Autodesk Fusion 360 part; units mm, degrees
(part 3 of 3)
  line L0 (23, 63.192) -> (0, 63.192)
  line L1 (0, 63.192) -> (0, 51.1685)
  line L2 (0, 51.1685) -> (23, 51.1685)
  line L3 (23, 51.1685) -> (23, 63.192)
  point P0 (22.9329, 63.145)
  point P1 (22.8659, 63.098)
  point P2 (22.799, 63.0511)
  point P3 (22.7322, 63.0043)
  point P4 (22.6656, 62.9575)
  point P5 (22.5991, 62.9107)
  point P6 (22.5326, 62.864)
  point P7 (22.4664, 62.8174)
  point P8 (22.4002, 62.7708)
  point P9 (22.3341, 62.7243)
  point P10 (22.2682, 62.6778)
  point P11 (22.2023, 62.6313)
  point P12 (22.1366, 62.585)
  point P13 (22.071, 62.5386)
  point P14 (22.0056, 62.4924)
  point P15 (21.9402, 62.4462)
  point P16 (21.875, 62.4)
  point P17 (21.8098, 62.3539)
  point P18 (21.7448, 62.3079)
  point P19 (21.6799, 62.2619)
  point P20 (21.6152, 62.216)
  point P21 (21.5505, 62.1702)
  point P22 (21.486, 62.1244)
  point P23 (21.4215, 62.0786)
  point P24 (21.3572, 62.033)
  point P25 (21.2931, 61.9874)
  point P26 (21.229, 61.9419)
  point P27 (21.165, 61.8964)
  point P28 (21.1012, 61.851)
  point P29 (21.0375, 61.8057)
  point P30 (20.9739, 61.7604)
  point P31 (20.9104, 61.7152)
  point P32 (20.847, 61.6701)
  point P33 (20.7837, 61.625)
  point P34 (20.7206, 61.58)
  point P35 (20.6576, 61.5351)
  point P36 (20.5947, 61.4902)
  point P37 (20.5319, 61.4455)
  point P38 (20.4692, 61.4008)
  point P39 (20.4066, 61.3561)
  point P40 (20.3442, 61.3116)
  point P41 (20.2819, 61.2671)
  point P42 (20.2197, 61.2227)
  point P43 (20.1576, 61.1783)
  point P44 (20.0956, 61.1341)
  point P45 (20.0337, 61.0899)
  point P46 (19.972, 61.0458)
  point P47 (19.9103, 61.0017)
  point P48 (19.8488, 60.9578)
  point P49 (19.7874, 60.9139)
  point P50 (19.7261, 60.8701)
  point P51 (19.6649, 60.8264)
  point P52 (19.6039, 60.7827)
  point P53 (19.5429, 60.7392)
  point P54 (19.4821, 60.6957)
  point P55 (19.4214, 60.6523)
  point P56 (19.3608, 60.609)
  point P57 (19.3003, 60.5657)
  point P58 (19.2399, 60.5226)
  point P59 (19.1796, 60.4795)
  point P60 (19.1195, 60.4365)
  point P61 (19.0595, 60.3936)
  point P62 (18.9995, 60.3508)
  point P63 (18.9397, 60.3081)
  point P64 (18.88, 60.2654)
  point P65 (18.8204, 60.2229)
  point P66 (18.761, 60.1804)
  point P67 (18.7016, 60.138)
  point P68 (18.6423, 60.0957)
  point P69 (18.5832, 60.0535)
  point P70 (18.5242, 60.0113)
  point P71 (18.4653, 59.9693)
  point P72 (18.4065, 59.9273)
  point P73 (18.3478, 59.8855)
  point P74 (18.2892, 59.8437)
  point P75 (18.2307, 59.802)
  point P76 (18.1724, 59.7604)
  point P77 (18.1141, 59.7189)
  point P78 (18.056, 59.6775)
  point P79 (17.9979, 59.6362)
  point P80 (17.94, 59.5949)
  point P81 (17.8822, 59.5538)
  point P82 (17.8245, 59.5127)
  point P83 (17.7669, 59.4718)
  point P84 (17.7094, 59.4309)
  point P85 (17.6521, 59.3902)
  point P86 (17.5948, 59.3495)
  point P87 (17.5376, 59.3089)
  point P88 (17.4806, 59.2684)
  point P89 (17.4236, 59.228)
  point P90 (17.3668, 59.1877)
  point P91 (17.3101, 59.1475)
  point P92 (17.2535, 59.1074)
  point P93 (17.197, 59.0674)
  point P94 (17.1406, 59.0275)
  point P95 (17.0843, 58.9877)
  point P96 (17.0281, 58.9479)
  point P97 (16.972, 58.9083)
  point P98 (16.916, 58.8688)
  point P99 (16.8601, 58.8293)
  point P100 (16.8044, 58.79)
  point P101 (16.7487, 58.7508)
  point P102 (16.6931, 58.7116)
  point P103 (16.6377, 58.6726)
  point P104 (16.5823, 58.6336)
  point P105 (16.5271, 58.5948)
  point P106 (16.472, 58.5561)
  point P107 (16.4169, 58.5174)
  point P108 (16.362, 58.4789)
  point P109 (16.3072, 58.4404)
  point P110 (16.2524, 58.4021)
  point P111 (16.1978, 58.3638)
  point P112 (16.1433, 58.3257)
  point P113 (16.0889, 58.2876)
  point P114 (16.0346, 58.2497)
  point P115 (15.9803, 58.2119)
  point P116 (15.9262, 58.1741)
  point P117 (15.8722, 58.1365)
  point P118 (15.8183, 58.099)
  point P119 (15.7645, 58.0615)
  point P120 (15.7108, 58.0242)
  point P121 (15.6572, 57.987)
  point P122 (15.6037, 57.9498)
  point P123 (15.5503, 57.9128)
  point P124 (15.4969, 57.8759)
  point P125 (15.4437, 57.8391)
  point P126 (15.3906, 57.8023)
  point P127 (15.3376, 57.7657)
  point P128 (15.2847, 57.7292)
  point P129 (15.2319, 57.6928)
  point P130 (15.1792, 57.6565)
  point P131 (15.1265, 57.6203)
  point P132 (15.074, 57.5842)
  point P133 (15.0216, 57.5482)
  point P134 (14.9692, 57.5123)
  point P135 (14.917, 57.4766)
  point P136 (14.8649, 57.4409)
  point P137 (14.8128, 57.4053)
  point P138 (14.7609, 57.3698)
  point P139 (14.709, 57.3345)
  point P140 (14.6573, 57.2992)
  point P141 (14.6056, 57.2641)
  point P142 (14.554, 57.229)
  point P143 (14.5026, 57.1941)
  point P144 (14.4512, 57.1592)
  point P145 (14.3999, 57.1245)
  point P146 (14.3487, 57.0899)
  point P147 (14.2976, 57.0553)
  point P148 (14.2466, 57.0209)
  point P149 (14.1957, 56.9866)
  point P150 (14.1448, 56.9524)
  point P151 (14.0941, 56.9183)
  point P152 (14.0435, 56.8843)
  point P153 (13.9929, 56.8504)
  point P154 (13.9424, 56.8167)
  point P155 (13.8921, 56.783)
  point P156 (13.8418, 56.7494)
  point P157 (13.7916, 56.7159)
  point P158 (13.7415, 56.6826)
  point P159 (13.6915, 56.6493)
  point P160 (13.6416, 56.6162)
  point P161 (13.5917, 56.5832)
  point P162 (13.542, 56.5502)
  point P163 (13.4923, 56.5174)
  point P164 (13.4428, 56.4847)
  point P165 (13.3933, 56.4521)
  point P166 (13.3439, 56.4196)
  point P167 (13.2946, 56.3872)
  point P168 (13.2454, 56.3549)
  point P169 (13.1962, 56.3227)
  point P170 (13.1472, 56.2906)
  point P171 (13.0982, 56.2587)
  point P172 (13.0494, 56.2268)
  point P173 (13.0006, 56.1951)
  point P174 (12.9519, 56.1634)
  point P175 (12.9032, 56.1319)
  point P176 (12.8547, 56.1004)
  point P177 (12.8062, 56.0691)
  point P178 (12.7579, 56.0379)
  point P179 (12.7096, 56.0068)
  point P180 (12.6614, 55.9758)
  point P181 (12.6133, 55.9449)
  point P182 (12.5652, 55.9141)
  point P183 (12.5173, 55.8834)
  point P184 (12.4694, 55.8528)
  point P185 (12.4216, 55.8223)
  point P186 (12.3739, 55.792)
  point P187 (12.3263, 55.7617)
  point P188 (12.2787, 55.7315)
  point P189 (12.2312, 55.7015)
  point P190 (12.1839, 55.6716)
  point P191 (12.1365, 55.6417)
  point P192 (12.0893, 55.612)
  point P193 (12.0422, 55.5824)
  point P194 (11.9951, 55.5529)
  point P195 (11.9481, 55.5235)
  point P196 (11.9012, 55.4942)
  point P197 (11.8543, 55.465)
  point P198 (11.8076, 55.4359)
  point P199 (11.7609, 55.4069)
  point P200 (11.7143, 55.378)
  point P201 (11.6678, 55.3493)
  point P202 (11.6213, 55.3206)
  point P203 (11.5749, 55.292)
  point P204 (11.5286, 55.2636)
  point P205 (11.4824, 55.2353)
  point P206 (11.4362, 55.207)
  point P207 (11.3902, 55.1789)
  point P208 (11.3442, 55.1509)
  point P209 (11.2982, 55.1229)
  point P210 (11.2524, 55.0951)
  point P211 (11.2066, 55.0674)
  point P212 (11.1609, 55.0398)
  point P213 (11.1153, 55.0123)
  point P214 (11.0697, 54.9849)
  point P215 (11.0242, 54.9576)
  point P216 (10.9788, 54.9305)
  point P217 (10.9334, 54.9034)
  point P218 (10.8882, 54.8764)
  point P219 (10.843, 54.8496)
  point P220 (10.7978, 54.8228)
  point P221 (10.7528, 54.7962)
  point P222 (10.7078, 54.7696)
  point P223 (10.6629, 54.7432)
  point P224 (10.618, 54.7168)
  point P225 (10.5732, 54.6906)
  point P226 (10.5285, 54.6645)
  point P227 (10.4839, 54.6384)
  point P228 (10.4393, 54.6125)
  point P229 (10.3948, 54.5867)
  point P230 (10.3503, 54.561)
  point P231 (10.306, 54.5354)
  point P232 (10.2616, 54.5099)
  point P233 (10.2174, 54.4845)
  point P234 (10.1732, 54.4592)
  point P235 (10.1291, 54.434)
  point P236 (10.0851, 54.4089)
  point P237 (10.0411, 54.384)
  point P238 (9.9972, 54.3591)
  point P239 (9.9534, 54.3343)
  point P240 (9.9096, 54.3096)
  point P241 (9.8659, 54.2851)
  point P242 (9.8222, 54.2606)
  point P243 (9.7786, 54.2363)
  point P244 (9.7351, 54.212)
  point P245 (9.6916, 54.1879)
  point P246 (9.6482, 54.1638)
  point P247 (9.6049, 54.1399)
  point P248 (9.5616, 54.116)
  point P249 (9.5184, 54.0923)
  point P250 (9.4753, 54.0686)
  point P251 (9.4322, 54.0451)
  point P252 (9.3892, 54.0217)
  point P253 (9.3462, 53.9983)
  point P254 (9.3033, 53.9751)
  point P255 (9.2604, 53.952)
  point P256 (9.2177, 53.929)
  point P257 (9.1749, 53.906)
  point P258 (9.1323, 53.8832)
  point P259 (9.0897, 53.8605)
  point P260 (9.0471, 53.8379)
  point P261 (9.0046, 53.8154)
  point P262 (8.9622, 53.793)
  point P263 (8.9198, 53.7706)
  point P264 (8.8775, 53.7484)
  point P265 (8.8353, 53.7263)
  point P266 (8.7931, 53.7043)
  point P267 (8.7509, 53.6824)
  point P268 (8.7088, 53.6606)
  point P269 (8.6668, 53.6389)
  point P270 (8.6248, 53.6173)
  point P271 (8.5829, 53.5958)
  point P272 (8.5411, 53.5744)
  point P273 (8.4993, 53.5531)
  point P274 (8.4575, 53.5319)
  point P275 (8.4158, 53.5108)
  point P276 (8.3742, 53.4898)
  point P277 (8.3326, 53.4689)
  point P278 (8.291, 53.4481)
  point P279 (8.2496, 53.4274)
  point P280 (8.2081, 53.4068)
  point P281 (8.1668, 53.3863)
  point P282 (8.1254, 53.3659)
  point P283 (8.0842, 53.3456)
  point P284 (8.043, 53.3253)
  point P285 (8.0018, 53.3052)
  point P286 (7.9607, 53.2852)
  point P287 (7.9196, 53.2653)
  point P288 (7.8786, 53.2455)
  point P289 (7.8376, 53.2258)
  point P290 (7.7967, 53.2062)
  point P291 (7.7559, 53.1867)
  point P292 (7.7151, 53.1673)
  point P293 (7.6743, 53.1479)
  point P294 (7.6336, 53.1287)
  point P295 (7.5929, 53.1096)
  point P296 (7.5523, 53.0906)
  point P297 (7.5117, 53.0717)
  point P298 (7.4712, 53.0528)
  point P299 (7.4308, 53.0341)
  point P300 (7.3903, 53.0155)
  point P301 (7.35, 52.9969)
  point P302 (7.3096, 52.9785)
  point P303 (7.2694, 52.9602)
  point P304 (7.2291, 52.9419)
  point P305 (7.1889, 52.9238)
  point P306 (7.1488, 52.9057)
  point P307 (7.1087, 52.8878)
  point P308 (7.0687, 52.8699)
  point P309 (7.0287, 52.8522)
  point P310 (6.9887, 52.8345)
  point P311 (6.9488, 52.8169)
  point P312 (6.9089, 52.7995)
  point P313 (6.8691, 52.7821)
  point P314 (6.8293, 52.7648)
  point P315 (6.7896, 52.7476)
  point P316 (6.7499, 52.7306)
  point P317 (6.7102, 52.7136)
  point P318 (6.6706, 52.6967)
  point P319 (6.6311, 52.6799)
  point P320 (6.5915, 52.6632)
  point P321 (6.5521, 52.6466)
  point P322 (6.5126, 52.6301)
  point P323 (6.4732, 52.6137)
  point P324 (6.4339, 52.5973)
  point P325 (6.3946, 52.5811)
  point P326 (6.3553, 52.565)
  point P327 (6.316, 52.5489)
  point P328 (6.2769, 52.533)
  point P329 (6.2377, 52.5172)
  point P330 (6.1986, 52.5014)
  point P331 (6.1595, 52.4858)
  point P332 (6.1205, 52.4702)
  point P333 (6.0815, 52.4547)
  point P334 (6.0425, 52.4394)
  point P335 (6.0036, 52.4241)
  point P336 (5.9647, 52.4089)
  point P337 (5.9259, 52.3938)
  point P338 (5.8871, 52.3788)
  point P339 (5.8483, 52.3639)
  point P340 (5.8096, 52.3491)
  point P341 (5.7709, 52.3344)
  point P342 (5.7323, 52.3198)
  point P343 (5.6936, 52.3053)
  point P344 (5.6551, 52.2908)
  point P345 (5.6165, 52.2765)
  point P346 (5.578, 52.2623)
  point P347 (5.5395, 52.2481)
  point P348 (5.5011, 52.2341)
  point P349 (5.4627, 52.2201)
  point P350 (5.4243, 52.2062)
  point P351 (5.386, 52.1924)
  point P352 (5.3477, 52.1788)
  point P353 (5.3094, 52.1652)
  point P354 (5.2712, 52.1517)
  point P355 (5.233, 52.1383)
  point P356 (5.1948, 52.1249)
  point P357 (5.1567, 52.1117)
  point P358 (5.1186, 52.0986)
  point P359 (5.0806, 52.0856)
  point P360 (5.0425, 52.0726)
  point P361 (5.0045, 52.0598)
  point P362 (4.9665, 52.047)
  point P363 (4.9286, 52.0344)
  point P364 (4.8907, 52.0218)
  point P365 (4.8528, 52.0093)
  point P366 (4.815, 51.9969)
  point P367 (4.7772, 51.9846)
  point P368 (4.7394, 51.9724)
  point P369 (4.7016, 51.9603)
  point P370 (4.6639, 51.9483)
  point P371 (4.6262, 51.9364)
  point P372 (4.5886, 51.9245)
  point P373 (4.5509, 51.9128)
  point P374 (4.5133, 51.9011)
  point P375 (4.4757, 51.8896)
  point P376 (4.4382, 51.8781)
  point P377 (4.4007, 51.8667)
  point P378 (4.3632, 51.8554)
  point P379 (4.3257, 51.8442)
  point P380 (4.2883, 51.8331)
  point P381 (4.2509, 51.8221)
  point P382 (4.2135, 51.8112)
  point P383 (4.1761, 51.8004)
  point P384 (4.1388, 51.7896)
  point P385 (4.1015, 51.779)
  point P386 (4.0642, 51.7684)
  point P387 (4.027, 51.758)
  point P388 (3.9898, 51.7476)
  point P389 (3.9526, 51.7373)
  point P390 (3.9154, 51.7271)
  point P391 (3.8783, 51.717)
  point P392 (3.8411, 51.707)
  point P393 (3.804, 51.6971)
  point P394 (3.767, 51.6873)
  point P395 (3.7299, 51.6776)
  point P396 (3.6929, 51.6679)
  point P397 (3.6559, 51.6584)
  point P398 (3.6189, 51.6489)
  point P399 (3.5819, 51.6395)
  point P400 (3.545, 51.6303)
  point P401 (3.5081, 51.6211)
  point P402 (3.4712, 51.612)
  point P403 (3.4344, 51.603)
  point P404 (3.3975, 51.5941)
  point P405 (3.3607, 51.5852)
  point P406 (3.3239, 51.5765)
  point P407 (3.2871, 51.5679)
  point P408 (3.2504, 51.5593)
  point P409 (3.2136, 51.5509)
  point P410 (3.1769, 51.5425)
  point P411 (3.1402, 51.5342)
  point P412 (3.1035, 51.526)
  point P413 (3.0669, 51.5179)
  point P414 (3.0302, 51.5099)
  point P415 (2.9936, 51.502)
  point P416 (2.957, 51.4942)
  point P417 (2.9205, 51.4865)
  point P418 (2.8839, 51.4788)
  point P419 (2.8474, 51.4713)
  point P420 (2.8108, 51.4638)
  point P421 (2.7743, 51.4565)
  point P422 (2.7378, 51.4492)
  point P423 (2.7014, 51.442)
  point P424 (2.6649, 51.4349)
  point P425 (2.6285, 51.4279)
  point P426 (2.5921, 51.421)
  point P427 (2.5557, 51.4142)
  point P428 (2.5193, 51.4075)
  point P429 (2.4829, 51.4009)
  point P430 (2.4466, 51.3943)
  point P431 (2.4102, 51.3879)
  point P432 (2.3739, 51.3815)
  point P433 (2.3376, 51.3752)
  point P434 (2.3013, 51.3691)
  point P435 (2.2651, 51.363)
  point P436 (2.2288, 51.357)
  point P437 (2.1926, 51.3511)
  point P438 (2.1563, 51.3453)
  point P439 (2.1201, 51.3396)
  point P440 (2.0839, 51.3339)
  point P441 (2.0477, 51.3284)
  point P442 (2.0115, 51.323)
  point P443 (1.9754, 51.3176)
  point P444 (1.9392, 51.3124)
  point P445 (1.9031, 51.3072)
  point P446 (1.867, 51.3021)
  point P447 (1.8309, 51.2972)
  point P448 (1.7948, 51.2923)
  point P449 (1.7587, 51.2875)
  point P450 (1.7226, 51.2828)
  point P451 (1.6865, 51.2782)
  point P452 (1.6505, 51.2737)
  point P453 (1.6144, 51.2692)
  point P454 (1.5784, 51.2649)
  point P455 (1.5424, 51.2607)
  point P456 (1.5064, 51.2565)
  point P457 (1.4704, 51.2525)
  point P458 (1.4344, 51.2485)
  point P459 (1.3984, 51.2447)
  point P460 (1.3624, 51.2409)
  point P461 (1.3265, 51.2372)
  point P462 (1.2905, 51.2337)
  point P463 (1.2545, 51.2302)
  point P464 (1.2186, 51.2268)
  point P465 (1.1827, 51.2235)
  point P466 (1.1468, 51.2203)
  point P467 (1.1108, 51.2172)
  point P468 (1.0749, 51.2142)
  point P469 (1.039, 51.2112)
  point P470 (1.0031, 51.2084)
  point P471 (0.9673, 51.2057)
  point P472 (0.9314, 51.2031)
  point P473 (0.8955, 51.2005)
  point P474 (0.8596, 51.1981)
  point P475 (0.8238, 51.1957)
  point P476 (0.7879, 51.1935)
  point P477 (0.7521, 51.1913)
  point P478 (0.7162, 51.1893)
  point P479 (0.6804, 51.1873)
  point P480 (0.6445, 51.1854)
  point P481 (0.6087, 51.1837)
  point P482 (0.5729, 51.182)
  point P483 (0.5371, 51.1804)
  point P484 (0.5012, 51.1789)
  point P485 (0.4654, 51.1776)
  point P486 (0.4296, 51.1763)
  point P487 (0.3938, 51.1751)
  point P488 (0.358, 51.174)
  point P489 (0.3222, 51.173)
  point P490 (0.2864, 51.1721)
  point P491 (0.2506, 51.1713)
  point P492 (0.2148, 51.1706)
  point P493 (0.179, 51.17)
  point P494 (0.1432, 51.1695)
  point P495 (0.1074, 51.1691)
  point P496 (0.0716, 51.1688)
  point P497 (0.0358, 51.1686)
  constraint horizontal L0
  constraint vertical L1
  constraint horizontal L2
  constraint vertical L3
revolve "回転1" add sketch "スケッチ1" angle 360 about axis through (0, 63.192, 0) along (0, -1, 0) contours S0 L0 L1
move_body "移動1" bodies 1 to x (1, 0, 0) y (0, 0, 1) z (0, -1, 0) at (0, 28.1685, -74.1685)
move_body "移動2" bodies 1 to x (1, 0, 0) y (0, -1, 0) z (0, 0, -1) at (0, 10.3371, -46)
sketch "スケッチ2" plane through (0, 0, 0) normal (0, 0, 1) x (1, 0, 0)
  circle A0 centre (0, 0) radius 23
  dimension "d2" = 46
  constraint coincident A0.centre origin
  measures "d2" diameter of A0
move_body "移動3" bodies 1 to x (1, 0, 0) y (0, 1, 0) z (0, 0, 1) at (0, 17.8315, 35.0234)
equation "d2 = ( 23 * 2 ) * 1 mm"
